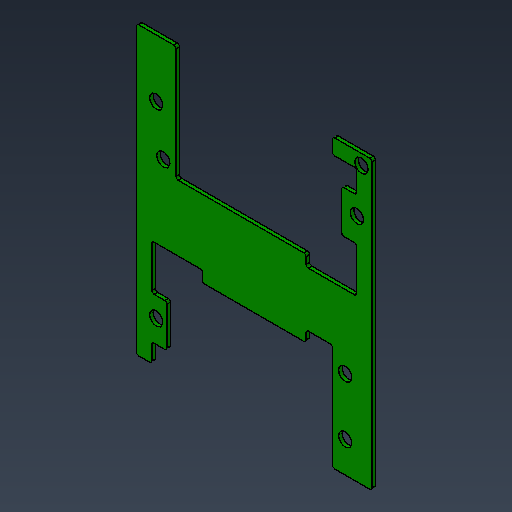
# Autodesk Inventor part: PCB_interface
Saved by Autodesk Inventor 2026.2 (Build 302298010, 298A)
## iProperties
Created: 2026-04-04
Part Number: PCB_interface
Material: Generic
Document SubType Name: Modeling
Designer: szymo
Density: 1 g/cm^3
Appearance: Default(2)
Author: szymo
Autodesk Inventor part; units mm, degrees
ref_plane "YZ Plane" through (0, 0, 0) normal (1, 0, 0) x (0, 1, 0)
ref_plane "XZ Plane" through (0, 0, 0) normal (0, 1, 0) x (-1, 0, 0)
ref_plane "XY Plane" through (0, 0, 0) normal (0, 0, 1) x (1, 0, 0)
sketch "Sketch1" plane through (0, 0, 0) normal (0, 0, 1) x (1, 0, 0)
  line L0 (-0.75, 14.7474) -> (-0.75, 16.5483) projected
  line L1 (-4.156, -4.2282) -> (-4.156, 0) projected
  line L2 (-0.75, 0) -> (-0.75, 9.8085) projected
  line L3 (1.35, 61.6927) -> (1.35, 16.5483) projected
  line L4 (1.35, 61.6927) -> (-7.856, 61.6927) projected
  line L5 (-7.856, -4.2282) -> (-7.856, 61.6927) projected
  line L6 (-4.156, 9.8085) -> (-4.156, 14.7474) projected
  line L7 (-0.75, 0) -> (-4.156, 0) projected
  line L8 (38.75, 42.531) -> (38.75, 52.3395) projected
  line L9 (38.75, 42.531) -> (42.15, 42.531) projected
  line L10 (42.15, 37.5922) -> (42.15, 42.531) projected
  line L11 (38.75, 37.5922) -> (42.15, 37.5922) projected
  line L12 (38.75, 35.7912) -> (38.75, 37.5922) projected
  line L13 (38.75, 35.7912) -> (36.65, 35.7912) projected
  line L14 (36.65, -4.2282) -> (36.65, 35.7912) projected
  line L15 (45.85, -4.2282) -> (36.65, -4.2282) projected
  line L16 (45.85, 61.0677) -> (45.85, -4.2282) projected
  line L17 (45.85, 61.0677) -> (36.65, 61.0677) projected
  line L18 (36.65, 57.3442) -> (36.65, 61.0677) projected
  line L19 (38.75, 57.3442) -> (36.65, 57.3442) projected
  line L20 (38.75, 56.3553) -> (38.75, 57.3442) projected
  line L21 (38.75, 56.3553) -> (42.15, 56.3553) projected
  line L22 (42.15, 52.3395) -> (42.15, 56.3553) projected
  line L23 (38.75, 52.3395) -> (42.15, 52.3395) projected
  line L24 (-0.75, 16.5483) -> (37.4, 16.5483)
  line L25 (37.4, 16.5483) -> (37.4, -5.0046)
  line L26 (37.4, -5.0046) -> (0, -5.0046)
  line L27 (0, -5.0046) -> (0, 11.1139)
  line L28 (0, 11.1139) -> (-3, 11.1139)
  line L29 (-3, 11.1139) -> (-3, 13.2925)
  line L30 (-3, 13.2925) -> (0, 13.2925)
  line L31 (0, 13.2925) -> (0, 16.5483)
  line L32 (5.5, 17.3718) -> (33.4, 17.3718)
  line L33 (33.4, 17.3718) -> (33.4, 16.5483)
  line L34 (33.4, 16.5483) -> (5.5, 16.5483)
  line L35 (5.5, 16.5483) -> (5.5, 17.3718)
  line L36 (33.4, -5.8282) -> (5.5, -5.8282)
  line L37 (5.5, -5.8282) -> (5.5, -5.0046)
  line L38 (5.5, -5.0046) -> (33.4, -5.0046)
  line L39 (33.4, -5.0046) -> (33.4, -5.8282)
  line L40 (32.5, 34.9677) -> (4.6, 34.9677)
  line L41 (4.6, 34.9677) -> (4.6, 35.7912)
  line L42 (4.6, 35.7912) -> (32.5, 35.7912)
  line L43 (32.5, 35.7912) -> (32.5, 34.9677)
  line L44 (4.6, 58.1677) -> (32.5, 58.1677)
  line L45 (32.5, 58.1677) -> (32.5, 57.3442)
  line L46 (32.5, 57.3442) -> (4.6, 57.3442)
  line L47 (4.6, 57.3442) -> (4.6, 58.1677)
  line L48 (38.75, 35.7912) -> (0.6, 35.7912)
  line L49 (0.6, 35.7912) -> (0.6, 57.3442)
  line L50 (0.6, 57.3442) -> (38.75, 57.3442)
  line L51 (38, 57.3442) -> (38, 41.2256)
  line L52 (38, 41.2256) -> (41, 41.2256)
  line L53 (41, 41.2256) -> (41, 39.047)
  line L54 (41, 39.047) -> (38, 39.047)
  line L55 (38, 39.047) -> (38, 35.7912)
  line L56 (1.35, 61.6927) -> (1.35, 34.1768)
  line L57 (1.25, 60.9677) -> (1.25, 34.8677)
  line L58 (1.25, 34.8677) -> (30.75, 34.8677)
  line L59 (1.25, 60.9677) -> (-7.756, 60.9677)
  line L60 (30.75, 34.8677) -> (30.75, 32.3677)
  line L61 (45.75, 32.8669) -> (45.75, -4.1282)
  line L62 (45.75, -4.1282) -> (36.75, -4.1282)
  line L63 (36.75, -4.1282) -> (36.75, 19.9718)
  line L64 (36.75, 19.9718) -> (30.75, 19.9718)
  line L65 (30.75, 19.9718) -> (30.75, 17.4718)
  line L66 (30.75, 17.4718) -> (27.7928, 17.4718)
  line L67 (27.7928, 17.4718) -> (7.25, 17.4718)
  line L68 (7.25, 17.4718) -> (7.25, 19.9718)
  line L69 (7.25, 19.9718) -> (-4.256, 19.9718)
  line L70 (-4.256, -4.1282) -> (-7.756, -4.1282)
  line L71 (-7.756, -4.1282) -> (-7.756, 60.9677)
  line L72 (30.75, 32.3677) -> (42.25, 32.3677)
  line L73 (42.1013, 60.9677) -> (45.75, 60.9677)
  line L74 (45.75, 60.9677) -> (45.75, 32.8669)
  line L75 (42.25, 32.3677) -> (42.25, 42.631)
  line L76 (42.25, 42.631) -> (38.85, 42.631)
  line L77 (38.85, 42.631) -> (38.85, 52.2395)
  line L78 (38.85, 52.2395) -> (42.25, 52.2395)
  line L79 (42.25, 52.2395) -> (42.25, 57.4442)
  line L80 (42.25, 57.4442) -> (36.75, 57.4442)
  line L81 (36.75, 57.4442) -> (36.75, 60.9677)
  line L82 (36.75, 60.9677) -> (42.1013, 60.9677)
  line L83 (-4.256, 19.9718) -> (-4.256, 9.7085)
  line L84 (-4.256, 9.7085) -> (-0.85, 9.7085)
  line L85 (-0.85, 9.7085) -> (-0.85, 0.1)
  line L86 (-0.85, 0.1) -> (-4.256, 0.1)
  line L87 (-4.256, 0.1) -> (-4.256, -4.1282)
  circle A0 centre (-3.25, 5.2167) radius 2.25 projected
  circle A1 centre (-3.253, 47.8715) radius 2.25 projected
  line L88 (42.25, 52.2395) -> (45.75, 52.2395)
  line L89 (-8.5, 61.6927) -> (-8.5, 48.0677) projected
  line L90 (-7.856, 61.0677) -> (-17, 61.0677) projected
  line L91 (-17, 56.3177) -> (-17, 61.0677) projected
  line L92 (-11.2, 56.3177) -> (-17, 56.3177) projected
  line L93 (-11.2, 56.3177) -> (-11.2, 48.0677) projected
  line L94 (-8.5, 48.0677) -> (-11.2, 48.0677) projected
  line L95 (-7.756, 60.9677) -> (-11.1, 60.9677)
  line L96 (-11.1, 60.9677) -> (-11.1, 48.1677)
  line L97 (-11.1, 48.1677) -> (-7.756, 48.1677)
  circle A2 centre (-1.65, 37.3004) radius 2.25 projected
  line L98 (-0.75, 9.8085) -> (-4.156, 9.8085) projected
  line L99 (-0.75, 14.7474) -> (-4.156, 14.7474) projected
  line L100 (-0.75, 16.5483) -> (1.35, 16.5483) projected
  line L101 (-4.156, -4.2282) -> (-7.856, -4.2282) projected
  circle A3 centre (43.3428, 58.5605) radius 2.25 projected
  circle A4 centre (39.65, 2.8902) radius 2.25 projected
  circle A5 centre (39.65, 15.8064) radius 2.25 projected
  circle A6 centre (42.3, 48.1395) radius 2.25 projected
  point P0 (0, 0)
  point P1 (2.1, 16.5483)
  point P2 (-0.75, -4.2282)
  point P3 (-0.75, -4.0158)
  point P4 (-0.85, 19.9718)
  dimension "d0" = 0.1
  dimension "d1" = 0.1
  dimension "d5" = 0.1
  dimension "d6" = 0.1
  dimension "d7" = 0.1
  dimension "d8" = 6
  dimension "d9" = 2.5
  dimension "d10" = 6
  dimension "d12" = 0.1
  dimension "d13" = 2.5
  dimension "d14" = 6
  dimension "d15" = 0.1
  dimension "d18" = 2.5
  dimension "d20" = 0.1
  dimension "d21" = 0.1
  dimension "d22" = 0.1
  dimension "d23" = 0.1
  dimension "d24" = 0.1
  dimension "d25" = 0.1
  dimension "d26" = 0.1
  dimension "d27" = 0.1
  dimension "d28" = 0.1
  dimension "d29" = 0.1
  dimension "d41" = 12.35
  dimension "d42" = 0.1
  dimension "d45" = 0.1
  dimension "d46" = 0
  dimension "d47" = 0.1
  dimension "d49" = 0.1
  constraints: 126 end point, 24 horizontal, 22 vertical, 13 perpendicular, 6 point on line, 1 parallel, 49 other
  measures "d0" distance between parallel lines of L58 L40
  measures "d5" distance between parallel lines of L16 L61
  measures "d6" distance between parallel lines of L15 L62
  measures "d8" distance between parallel lines of L63 L65
  measures "d9" distance between parallel lines of L66 L64
  measures "d10" distance between parallel lines of L63 L60
  measures "d12" distance between parallel lines of L32 L66
  measures "d13" distance between parallel lines of L69 L67
  measures "d14" distance between parallel lines of L57 L68
  measures "d18" distance between parallel lines of L58 L72
  measures "d20" distance between parallel lines of L17 L82
  measures "d21" distance between parallel lines of L18 L81
  measures "d22" distance between parallel lines of L19 L80
  measures "d23" distance between parallel lines of L22 L79
  measures "d24" distance between parallel lines of L23 L78
  measures "d25" distance between parallel lines of L8 L77
  measures "d26" distance between parallel lines of L76 L9
  measures "d27" distance between parallel lines of L87 L6
  measures "d28" distance between parallel lines of L86 L7
  measures "d29" distance between parallel lines of L0 L85
  measures "d41" distance between parallel lines of L57 L96
  measures "d42" distance between parallel lines of L96 L93
  measures "d45" distance between parallel lines of L97 L94
  measures "d46" distance between parallel lines of L78 L88
  measures "d47" distance between parallel lines of L98 L84
  measures "d49" distance from line of L95 L91.end
extrude "Extrusion1" add sketch "Sketch1" along normal blind 0.8 contours A2 | L69 L83 L84 L85 L86 L87 L70 L71 L59 L57 L50 L49 L48 L58 L3 | L3 L58 L60 L72 L14 L64 L65 L66 L67 L68 L69 | A5 | A4 | L14 L72 L75 L76 L77 L78 L88 L74 L61 L62 L25 L24 L63 L64 | L24 L25 L62 L63 | L48 L49 L50 L57 | L88 L79 A3 L80 L81 L82 L73 L74 | L79 L80 A3 | A0 | A1 | A6 picked at (43.9565, 59.311)
hole "Hole1" at (-3.253, 47.8715, 0) at (-3.25, 5.2167, 0) at (-1.65, 37.3004, 0) at (39.65, 15.8064, 0) at (39.65, 2.8902, 0) at (42.3, 48.1395, 0) at (43.3428, 58.5605, 0) direction (0, 0, 1) diameter 3 end through all
fillet "Fillet1" radius 0.5 28 edges at (30.75, 32.3677, 0.4) (30.75, 34.8677, 0.4) (42.25, 32.3677, 0.4) (42.25, 42.631, 0.4) (38.85, 42.631, 0.4) (38.85, 52.2395, 0.4) (42.25, 52.2395, 0.4) (42.25, 57.4442, 0.4) (36.75, 57.4442, 0.4) (36.75, 60.9677, 0.4) (45.75, 60.9677, 0.4) (45.75, -4.1282, 0.4) (36.75, -4.1282, 0.4) (36.75, 19.9718, 0.4) (30.75, 19.9718, 0.4) (30.75, 17.4718, 0.4) (7.25, 17.4718, 0.4) (7.25, 19.9718, 0.4) (-4.256, 19.9718, 0.4) (-4.256, 9.7085, 0.4) (-0.85, 9.7085, 0.4) (-0.85, 0.1, 0.4) (-4.256, 0.1, 0.4) (-4.256, -4.1282, 0.4) (-7.756, -4.1282, 0.4) (1.25, 60.9677, 0.4) (1.25, 34.8677, 0.4) (-7.756, 60.9677, 0.4)
equation "\"d9\" = d18"
equation "\"d13\" = d18"
body "Solid1"
